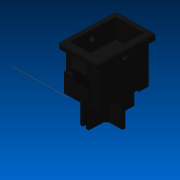
# Autodesk Inventor part: Arcolectric H8550VB Rocker Switch Housing
Saved by Autodesk Inventor 2016 (Build 200138000, 138)
## iProperties
Created: 2012-08-10
Material: Nylon 6/6
Document SubType Name: Modeling
Designer: sdarley
Density: 1.13 g/cm^3
Project: Rocker Switch - Arcolectric H8550VB
Description: Arcolectric H8550VB Rocker Switch Housing
Vendor: Arcolectric
Stock Number: H8550VB
Appearance: Black Control Joints
Author: sdarley
Title: Arcolectric H8550VB Rocker Switch Housing
Revision Number: 1
Autodesk Inventor part; units mm, degrees
ref_plane "YZ Plane" through (0, 0, 0) normal (1, 0, 0) x (0, 1, 0)
ref_plane "XZ Plane" through (0, 0, 0) normal (0, 1, 0) x (-1, 0, 0)
ref_plane "XY Plane" through (0, 0, 0) normal (0, 0, 1) x (1, 0, 0)
sketch "Sketch1" plane through (0, 0, 0) normal (0, 1, 0) x (-1, 0, 0)
  line L0 (7.475, 10.475) -> (-7.475, 10.475)
  line L1 (-7.475, 10.475) -> (-7.475, -10.475)
  line L2 (-7.475, -10.475) -> (7.475, -10.475)
  line L3 (7.475, -10.475) -> (7.475, 10.475)
  line L4 (7.475, 10.475) -> (-7.475, -10.475) construction
  line L5 (-7.475, 10.475) -> (7.475, -10.475) construction
  line L6 (5.25, 8.25) -> (-5.25, 8.25)
  line L7 (-5.25, 8.25) -> (-5.25, -8.25)
  line L8 (-5.25, -8.25) -> (5.25, -8.25)
  line L9 (5.25, -8.25) -> (5.25, 8.25)
  line L10 (5.25, 8.25) -> (-5.25, -8.25) construction
  line L11 (-5.25, 8.25) -> (5.25, -8.25) construction
  point P0 (0, 0)
  dimension "d0" = 14.95
  dimension "d1" = 20.95
  dimension "d2" = 10.5
  dimension "d3" = 16.5
  constraints: 24 end point, 4 midpoint, 4 parallel, 2 horizontal, 2 perpendicular
  measures "d0" distance of L2.end L1.end
  measures "d1" distance of L1.end L0.end
  measures "d2" distance of L8.end L7.end
  measures "d3" distance of L7.end L6.end
extrude "Extrusion1" add sketch "Sketch1" along normal blind 2
sketch "Sketch2" plane through (0, 0, 0) normal (0, -1, 0) x (1, 0, 0)
  line L0 (-5.25, -8.25) -> (-5.25, 8.25) projected
  line L1 (-5.25, 8.25) -> (5.25, 8.25) projected
  line L2 (5.25, 8.25) -> (5.25, -8.25) projected
  line L3 (5.25, -8.25) -> (-5.25, -8.25) projected
  line L4 (-6.4, -9.175) -> (6.4, -9.175)
  line L5 (6.4, -9.175) -> (6.4, 9.175)
  line L6 (6.4, 9.175) -> (-6.4, 9.175)
  line L7 (-6.4, 9.175) -> (-6.4, -9.175)
  line L8 (-6.4, -9.175) -> (6.4, 9.175) construction
  line L9 (6.4, -9.175) -> (-6.4, 9.175) construction
  point P0 (0, 0)
  dimension "d6" = 12.8
  dimension "d7" = 18.35
  constraints: 12 end point, 2 midpoint, 2 parallel, 1 horizontal, 1 perpendicular
  measures "d6" distance of L6.end L5.end
  measures "d7" distance of L5.end L4.end
extrude "Extrusion2" add sketch "Sketch2" along normal blind 14
sketch "Sketch3" plane through (0, -14, 0) normal (0, -1, 0) x (1, 0, 0)
  line L0 (-5.25, 8.25) -> (5.25, 8.25) projected
  line L1 (5.25, 8.25) -> (5.25, -8.25) projected
  line L2 (5.25, -8.25) -> (-5.25, -8.25) projected
  line L3 (-5.25, -8.25) -> (-5.25, 8.25) projected
  point P0 (0, 0)
extrude "Extrusion3" add sketch "Sketch3" against normal blind 9
sketch "Sketch4" plane through (6.4, 0, 9.175) normal (1, 0, 0) x (0, 0, -1)
  circle A0 centre (9.175, -1) radius 1
  line L0 (-1.3, 0) -> (19.65, 0) projected
  point P0 (9.175, 0)
  point P1 (9.175, 0)
  dimension "d12" = 2
  constraints: 1 centre point, 1 midpoint, 1 tangent, 1 vertical alignment
  measures "d12" diameter of A0
extrude "Extrusion4" cut sketch "Sketch4" against normal through all
sketch "Sketch5" plane through (-6.4, -14, -9.175) normal (-1, 0, 0) x (0, 0, 1)
  line L0 (0, 14) -> (0.65, 14)
  line L1 (0.65, 14) -> (0.65, 6.75)
  line L2 (0.65, 6.75) -> (0, 6.75)
  line L3 (0, 6.75) -> (0, 14)
  line L4 (18.35, 14) -> (17.7, 14)
  line L5 (17.7, 14) -> (17.7, 6.75)
  line L6 (17.7, 6.75) -> (18.35, 6.75)
  line L7 (18.35, 6.75) -> (18.35, 14)
  dimension "d15" = 7.25
  dimension "d17" = 17.05
  constraints: 16 end point, 4 parallel, 2 horizontal, 2 perpendicular, 1 collinear, 1 horizontal alignment
  measures "d15" distance between parallel lines of L2 L0
  measures "d17" distance between parallel lines of L5 L1
extrude "Extrusion5" cut sketch "Sketch5" against normal through all
sketch "Sketch6" plane through (0, -14, 0) normal (0, -1, 0) x (1, 0, 0)
  line L0 (6.4, -9.175) -> (6.4, 9.175) projected
  line L1 (6.4, 9.175) -> (-6.4, 9.175) projected
  line L2 (-6.4, -9.175) -> (6.4, -9.175) projected
  line L3 (-6.4, 9.175) -> (-6.4, -9.175) projected
  line L4 (6.4, -0.175) -> (6.4, 0.825)
  line L5 (-6.4, 0.825) -> (-6.4, -0.175)
  line L6 (-0.5, 9.175) -> (0.5, 9.175)
  line L7 (0.5, -9.175) -> (-0.5, -9.175)
  line L8 (6.4, 0.825) -> (1.3077, 0.825)
  line L9 (-1.3077, 0.825) -> (-6.4, 0.825)
  line L10 (-0.5, -9.175) -> (-0.5, -0.9827)
  line L11 (-0.5, 1.6327) -> (-0.5, 9.175)
  line L12 (0.5, 9.175) -> (0.5, 1.6327)
  line L13 (0.5, -0.9827) -> (0.5, -9.175)
  line L14 (-6.4, -0.175) -> (-1.3077, -0.175)
  line L15 (1.3077, -0.175) -> (6.4, -0.175)
  arc A0 (-0.5, 1.6327) -> (-1.3077, 0.825) centre (0, 0.325) ccw
  arc A1 (1.3077, 0.825) -> (0.5, 1.6327) centre (0, 0.325) ccw
  arc A2 (-1.3077, -0.175) -> (-0.5, -0.9827) centre (0, 0.325) ccw
  arc A3 (0.5, -0.9827) -> (1.3077, -0.175) centre (0, 0.325) ccw
  point P0 (0, 0)
  point P1 (0, 9.175)
  point P2 (0, 9.175)
  point P3 (0, 9.175)
  point P4 (-6.4, 0.325)
  point P5 (0, 0.325)
  point P6 (0, -9.175)
  point P7 (0, -9.175)
  dimension "d32" = 9
  dimension "d33" = 1
  dimension "d34" = 1
  dimension "d36" = 1.4
  constraints: 24 end point, 10 parallel, 8 point on circle, 6 midpoint, 6 vertical alignment, 5 horizontal alignment, 4 centre point, 4 perpendicular, 4 point on line, 3 horizontal, 2 coincident
  measures "d32" distance between parallel lines of L2 L14
  measures "d33" distance between parallel lines of L9 L14
  measures "d34" distance between parallel lines of L12 L11
  measures "d36" radius of A1
extrude "Extrusion6" add sketch "Sketch6" along normal blind 9 contours L15 A3 L13 L2 L10 A2 L14 L3 L9 A0 L11 L1 L12 A1 L8 L0
sketch "Sketch7" plane through (6.4, -7.25, -9.175) normal (0, 0, -1) x (-1, 0, 0)
  line L0 (12.8, -6.75) -> (0, -6.75) projected
  line L1 (0, 0) -> (3.7, 0)
  line L2 (3.7, 0) -> (3.7, -6.75)
  line L3 (3.7, -6.75) -> (0, -6.75)
  line L4 (0, -6.75) -> (0, 0)
  point P0 (6.4, 7.25)
  dimension "d25" = 3.7
  constraints: 8 end point, 2 parallel, 1 horizontal, 1 perpendicular, 1 point on line
  measures "d25" distance between parallel lines of L4 L2
extrude "Extrusion7" cut sketch "Sketch7" against normal up to surface (0.65 mm away)
mirror "Mirror1" about plane through (0, 0, 0) normal (0, 0, 1) of "Extrusion7"
sketch "Sketch8" plane through (-0.5, -14, 1.6327) normal (-1, 0, 0) x (0, 0, 1)
  line L0 (0, 0) -> (7.5423, 0) projected
  line L1 (7.5423, -9) -> (5.4923, -9)
  line L2 (5.4923, -9) -> (5.4923, -6.9)
  line L3 (5.4923, -6.9) -> (7.5423, -6.9)
  line L4 (7.5423, -6.9) -> (7.5423, -9)
  line L5 (-10.8077, 0) -> (-10.8077, -9) projected
  point P0 (-1.6327, 14)
  dimension "d37" = 16.3
  dimension "d38" = 6.9
  constraints: 8 end point, 2 parallel, 1 horizontal, 1 perpendicular
  measures "d37" distance between parallel lines of L2 L5
  measures "d38" distance between parallel lines of L3 L0
extrude "Extrusion8" cut sketch "Sketch8" against normal through all
sketch "Sketch9" plane through (0, 0, 0) normal (1, 0, 0) x (0, 1, 0)
  line L0 (0, -10.475) -> (0, 10.475) projected
  line L1 (-7.25, 8.525) -> (0, 8.525) projected
  line L2 (-7.25, 9.175) -> (-7.25, 8.525) projected
  line L3 (-7.25, 9.175) -> (-14, 9.175) projected
  line L4 (-14, 1.6327) -> (-14, 9.175) projected
  line L5 (0, 8.925) -> (-4, 9.225)
  line L6 (-4, 9.225) -> (-7.25, 8.925)
  arc A0 (-3.9, 10.225) -> (0, 9.725) centre (-0.0802, 24.5597) ccw
  line L7 (-3.9, 10.225) -> (-8.3, 9.175)
  point P0 (0, 0)
  dimension "d41" = 0.7
  dimension "d42" = 0.4
  dimension "d43" = 4
  dimension "d44" = 3.9
  dimension "d45" = 8.3
  dimension "d46" = 0.8
  dimension "d47" = 1
  dimension "d48" = 0.75
  constraints: 6 end point, 4 point on line, 2 point on circle, 1 centre point, 1 horizontal alignment
  measures "d41" distance from line of L5.end L1
  measures "d42" distance from line of L5.start L1
  measures "d43" distance from line of L5.end L0
  measures "d44" distance from line of L7.start L0
  measures "d45" distance from line of L7.end L0
  measures "d46" distance of L5.start A0.end
  measures "d47" vertical distance of L7.start L5.end
  measures "d48" distance edge to line of A0 L5
extrude "Extrusion9" add sketch "Sketch9" along normal mid plane 5.4 contours L5 L6 L2 L3 L7 A0 L0
sketch "Sketch10" plane through (-2.7, 0, 0) normal (-1, 0, 0) x (0, 0, 1)
  arc A0 (9.725, 0) -> (10.225, -3.9) centre (24.5597, -0.0802) ccw projected
  line L0 (8.925, 0) -> (9.725, 0) projected
  line L1 (9.7357, -0.65) -> (9.5253, -0.785)
  line L2 (9.5253, -0.785) -> (9.7474, -0.8997)
  point P0 (0, 0)
  dimension "d52" = 0.25
  dimension "d54" = 0.25
  dimension "d55" = 0.65
  dimension "d56" = 60
  constraints: 4 end point, 2 point on circle
  measures "d52" distance of L1.start L2.end
  measures "d54" distance of L1.start L1.end
  measures "d55" distance from line of L1.start L0
  measures "d56" angle of L2 L1
extrude "Extrusion10" cut sketch "Sketch10" against normal through all
pattern_circular "Circular Pattern1" count 6 over 11 about axis through (0, -0.0802, 24.5597) along (-1, 0, 0) of "Extrusion10"
mirror "Mirror2" about plane through (0, 0, 0) normal (0, 0, 1) of "Extrusion9", "Extrusion10", "Circular Pattern1"
sketch "Sketch11" plane through (0, 0, 0) normal (0, -1, 0) x (1, 0, 0)
  line L0 (-6.4, 8.525) -> (6.4, 8.525) projected
  line L1 (6.4, 8.525) -> (6.4, 0) projected
  line L2 (7.475, -10.475) -> (-7.475, -10.475) projected
  arc A0 (6.4, 6.925) -> (6.4, 7.575) centre (6.374, 7.25) ccw
  line L3 (6.4, 7.575) -> (6.4, 6.925)
  point P0 (0, 0)
  dimension "d62" = 0.95
  dimension "d63" = 0.65
  dimension "d64" = 0.3
  constraints: 2 end point, 2 point on circle, 2 point on line, 1 centre point, 1 perpendicular
  measures "d62" distance from line of L0 L3.start
  measures "d63" distance of L3.start L3.end
  measures "d64" distance edge to line of A0 L1
extrude "Extrusion11" add sketch "Sketch11" along normal blind 5.4
fillet "Fillet1" radius 0.3 1 edges at (6.7, -5.4, 7.25)
mirror "Mirror3" about plane through (0, 0, 0) normal (1, 0, 0) of "Extrusion11", "Fillet1"
mirror "Mirror4" about plane through (0, 0, 0) normal (0, 0, 1) of "Extrusion11", "Fillet1", "Mirror3"
sketch "Sketch12" plane through (-6.4, -1, 0) normal (-1, 0, 0) x (0, 0, 1)
  line L0 (-9.175, -6.25) -> (-9.175, -13) projected
  line L1 (-0.175, -13) -> (-9.175, -13) projected
  line L2 (9.175, -13) -> (0.825, -13) projected
  line L3 (9.175, -6.25) -> (9.175, -13) projected
  line L4 (-4.975, -13) -> (-3.125, -13)
  line L5 (-3.125, -13) -> (-3.125, -12.35)
  line L6 (-3.125, -12.35) -> (-4.975, -12.35)
  line L7 (-4.975, -12.35) -> (-4.975, -13)
  line L8 (3.975, -13) -> (5.825, -13)
  line L9 (5.825, -13) -> (5.825, -12.35)
  line L10 (5.825, -12.35) -> (3.975, -12.35)
  line L11 (3.975, -12.35) -> (3.975, -13)
  dimension "d68" = 1.85
  dimension "d70" = 4.2
  dimension "d71" = 0.65
  dimension "d72" = 3.35
  dimension "d73" = 1.85
  constraints: 16 end point, 4 parallel, 2 horizontal, 2 perpendicular, 2 point on line, 1 horizontal alignment
  measures "d68" distance between parallel lines of L5 L7
  measures "d70" distance between parallel lines of L0 L7
  measures "d71" distance between parallel lines of L1 L6
  measures "d72" distance between parallel lines of L3 L9
  measures "d73" distance of L9.end L10.end
extrude "Extrusion12" cut sketch "Sketch12" against normal blind 5.5
mirror "Mirror5" about plane through (0, 0, 0) normal (1, 0, 0) of "Extrusion12"
fillet "Fillet2" radius 1 8 edges at (-7.475, 1, -10.475) (7.475, 1, -10.475) (7.475, 1, 10.475) (-7.475, 1, 10.475) (0, 2, -10.475) (7.475, 2, 0) (0, 2, 10.475) (-7.475, 2, 0)
fillet "Fillet3" radius 0.1 26 edges at (0, -3.9, -10.225) (0, -3.711, -10.176) (0, -3.1561, -10.0472) (0, -2.5968, -9.9398) (0, -2.9112, -9.9974) (0, -3.4681, -10.1168) (0, -2.3501, -9.8995) (0, -2.0337, -9.854) (0, -1.7856, -9.8231) (0, -1.4677, -9.7898) (0, -1.2186, -9.7685) (0, -0.65, -9.7357) (0, -0.8997, -9.7474) (0, -0.65, 9.7357) (0, -0.8997, 9.7474) (0, -1.2186, 9.7685) (0, -1.4677, 9.7898) (0, -1.7856, 9.8231) (0, -2.0337, 9.854) (0, -2.3501, 9.8995) (0, -2.5968, 9.9398) (0, -2.9112, 9.9974) (0, -3.1561, 10.0472) (0, -3.4681, 10.1168) (0, -3.711, 10.176) (0, -3.9, 10.225)
fillet "Fillet4" radius 0.05 12 edges at (0, -0.785, -9.5253) (0, -1.3616, -9.5635) (0, -1.9364, -9.6237) (0, -2.5083, -9.706) (0, -3.0768, -9.8101) (0, -3.6408, -9.936) (0, -3.6408, 9.936) (0, -3.0768, 9.8101) (0, -2.5083, 9.706) (0, -1.9364, 9.6237) (0, -1.3616, 9.5635) (0, -0.785, 9.5253)
equation "\"d34\" = d33"
equation "\"d54\" = d52"
equation "\"d73\" = d68"
equation "\"d31\" = d30"
equation "\"d30\" = 1"
body "Solid1"
